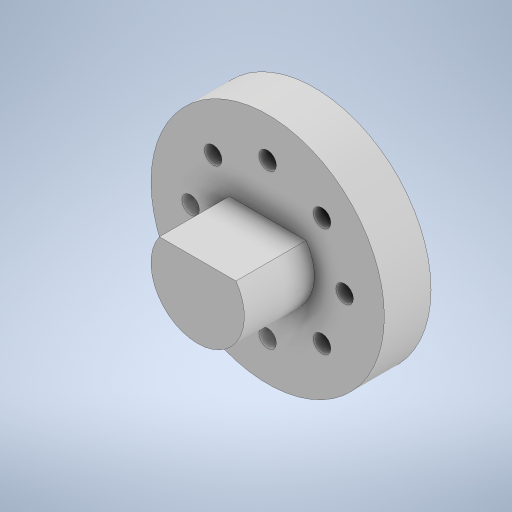
# Autodesk Inventor part: Part2
Saved by Autodesk Inventor 2024 (Build 280153000, 153)
## iProperties
Created: 2025-08-09
Part Number: Part2
Material: Generic
Document SubType Name: Modeling
Designer: albah
Density: 1 g/cm^3
Appearance: Default
Author: albah
Autodesk Inventor part; units mm, degrees
ref_plane "YZ Plane" through (0, 0, 0) normal (1, 0, 0) x (0, 1, 0)
ref_plane "XZ Plane" through (0, 0, 0) normal (0, 1, 0) x (-1, 0, 0)
ref_plane "XY Plane" through (0, 0, 0) normal (0, 0, 1) x (1, 0, 0)
sketch "Sketch1" plane through (0, 0, 0) normal (0, 0, 1) x (1, 0, 0)
  circle A0 centre (0, 0) radius 10
  line L0 (0, 0) -> (0, 6.6)
  circle A1 centre (0, 6.6) radius 0.75
  circle A2 centre (0, 0) radius 4
  line L1 (-3.2829, 2.2854) -> (3.2829, 2.2854)
  circle A3 centre (-4.6669, 4.6669) radius 0.75
  circle A4 centre (-6.6, 0) radius 0.75
  circle A5 centre (-4.6669, -4.6669) radius 0.75
  circle A6 centre (0, -6.6) radius 0.75
  circle A7 centre (4.6669, -4.6669) radius 0.75
  circle A8 centre (6.6, 0) radius 0.75
  circle A9 centre (4.6669, 4.6669) radius 0.75
  dimension "d0" = 20
  dimension "d1" = 6.6
  dimension "d2" = 1.5
  dimension "d3" = 8
  dimension "d4" = 2.2854
  dimension "d11" = 360
  constraints: 12 coincident, 10 centre point, 4 end point, 2 point on circle, 1 horizontal, 1 vertical, 31 other
  measures "d0" diameter of A0
  measures "d1" distance of L0.start L0.end
  measures "d2" diameter of A1
  measures "d3" diameter of A2
  measures "d4" distance from line of point (0, 0) L1
extrude "Extrusion1" add sketch "Sketch1" along normal blind 4 contours A0 | L1 A2 L0 | L0 A2 L1
extrude "Extrusion2" add sketch "Sketch1" along normal blind 10 contours L1 A2
body "Solid1"
